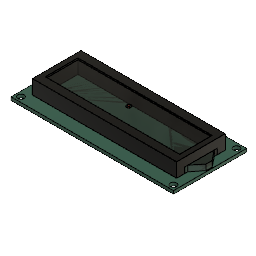
OTT Servo Tester Enclosure (Autodesk Fusion 360 archive; units mm, degrees)
design "1602 LCD Simplified Model"
Autodesk Fusion 360 part; units mm, degrees
sketch "LCD PCB" plane through (0, 0, 0) normal (0, 0, 1) x (1, 0, 0) in component "LCD PCB"
  line L0 (-40, 18) -> (40, 18)
  line L1 (40, 18) -> (40, -18)
  line L2 (40, -18) -> (-40, -18)
  line L3 (-40, -18) -> (-40, 18)
  line L4 (-40, 18) -> (40, -18) construction
  line L5 (40, 18) -> (-40, -18) construction
  line L6 (0, 1.75) -> (0, 22.5)
  line L7 (1.75, 0) -> (22.5, 0)
  point P0 (-37.5, 15.5)
  point P1 (37.5, 15.5)
  point P2 (-37.5, -15.5)
  point P3 (37.5, -15.5)
  point P4 (-32, 15.46)
  point P5 (-29.46, 15.46)
  point P6 (-26.92, 15.46)
  point P7 (-24.38, 15.46)
  point P8 (-21.84, 15.46)
  point P9 (-19.3, 15.46)
  point P10 (-16.76, 15.46)
  point P11 (-14.22, 15.46)
  point P12 (-11.68, 15.46)
  point P13 (-9.14, 15.46)
  point P14 (-6.6, 15.46)
  point P15 (-4.06, 15.46)
  point P16 (-1.52, 15.46)
  point P17 (1.02, 15.46)
  point P18 (3.56, 15.46)
  point P19 (6.1, 15.46)
  dimension "d1" = 80
  dimension "d2" = 36
  dimension "d3" = 2.5
  dimension "d4" = 2.5
  dimension "d5" = 8
  dimension "d6" = 2.54
  dimension "d9" = 2.54
  dimension "d10" = 0
  constraint horizontal L0
  constraint perpendicular L0 L1
  constraint parallel L0 L2
  constraint parallel L1 L3
  constraint coincident L4 origin
  constraint coincident L5 origin
  constraint symmetric P0 L6 P1
  constraint symmetric P0 L7 P2
  constraint symmetric P1 L7 P3
  measures "d1" distance of L1.end L2.end
  measures "d2" distance of L0.end L1.end
  measures "d3" distance of L0 P0
  measures "d4" distance of L3 P0
  measures "d5" distance of L3 P4
  measures "d6" distance of L0 P4
extrude "Extrude1" add sketch "LCD PCB" against normal blind 1.6 makes body 1 in component "LCD PCB"
hole "Hole1" at (-37.5, 15.5, 0) at (-37.5, -15.5, 0) at (37.5, -15.5, 0) at (37.5, 15.5, 0) direction (0, 0, -1) diameter 3.1 end up to surface (1.6 mm away) bodies 1 in component "LCD PCB"
hole "Hole2" at (6.1, 15.46, 0) at (3.56, 15.46, 0) at (1.02, 15.46, 0) at (-1.52, 15.46, 0) at (-4.06, 15.46, 0) at (-6.6, 15.46, 0) at (-9.14, 15.46, 0) at (-11.68, 15.46, 0) at (-14.22, 15.46, 0) at (-16.76, 15.46, 0) at (-19.3, 15.46, 0) at (-21.84, 15.46, 0) at (-24.38, 15.46, 0) at (-26.92, 15.46, 0) at (-29.46, 15.46, 0) at (-32, 15.46, 0) direction (0, 0, -1) diameter 1 depth 1.6 tip angle 180 bodies 1 in component "LCD PCB"
sketch "Bezel" plane through (0, 0, 0) normal (0, 0, 1) x (1, 0, 0) in component "LCD Bezel"
  line L0 (35.5, 12) -> (-35.5, 12)
  line L1 (-35.5, 12) -> (-35.5, -12)
  line L2 (-35.5, -12) -> (35.5, -12)
  line L3 (35.5, -12) -> (35.5, 12)
  line L4 (35.5, 12) -> (-35.5, -12) construction
  line L5 (-35.5, 12) -> (35.5, -12) construction
  line L6 (-33, 8) -> (33, 8)
  line L7 (33, 8) -> (33, -8)
  line L8 (33, -8) -> (-33, -8)
  line L9 (-33, -8) -> (-33, 8)
  line L10 (-33, 8) -> (33, -8) construction
  line L11 (33, 8) -> (-33, -8) construction
  dimension "d19" = 71
  dimension "d20" = 24
  dimension "d21" = 66
  dimension "d22" = 16
  constraint horizontal L0
  constraint perpendicular L0 L1
  constraint parallel L0 L2
  constraint parallel L1 L3
  constraint coincident L4 origin
  constraint coincident L5 origin
  constraint horizontal L6
  constraint perpendicular L6 L7
  constraint parallel L6 L8
  constraint parallel L7 L9
  constraint coincident L10 origin
  constraint coincident L11 origin
  measures "d19" distance of L1.end L2.end
  measures "d20" distance of L0.end L1.end
  measures "d21" distance of L7.end L8.end
  measures "d22" distance of L6.end L7.end
extrude "Extrude1'" add sketch "Bezel" along normal blind 7 separate body makes body 2 in component "LCD Bezel"
sketch "LCD Glass" plane through (0, 0, 7) normal (0, 0, 1) x (-1, 0, 0) in component "LCD Glass"
  line L0 (-33, 8) -> (33, 8)
  line L1 (33, 8) -> (33, -8)
  line L2 (33, -8) -> (-33, -8)
  line L3 (-33, -8) -> (-33, 8)
  line L4 (-35.5, 12) -> (-35.5, -12)
  line L5 (-35.5, -12) -> (35.5, -12)
  line L6 (35.5, -12) -> (35.5, 12)
  line L7 (35.5, 12) -> (-35.5, 12)
  line L8 (-35.5, 0) -> (-35.5, -6.5) construction
  line L9 (-35.5, -6.5) -> (-39.5, -1.5)
  line L10 (-39.5, -1.5) -> (-39.5, 0)
  line L11 (-1.75, 0) -> (-22.5, 0)
  line L12 (-40, -18) -> (-40, 18)
  line L13 (-35.5, 0) -> (-35.5, 6.5) construction
  line L14 (-35.5, 6.5) -> (-39.5, 1.5)
  line L15 (-39.5, 1.5) -> (-39.5, 0)
  line L16 (-35.5, -6.5) -> (-35.5, -8)
  line L17 (33, -8) -> (33, 8)
  line L18 (-35.5, 8) -> (-35.5, 6.5)
  line L19 (-35.5, 8) -> (33, 8)
  line L20 (33, -8) -> (-35.5, -8)
  line L21 (-35.5, -6.5) -> (-35.5, -8)
  circle A0 centre (0, 0) radius 1
  line L22 (0, -1) -> (0, 1)
  line L23 (1, 0) -> (-1, 0)
  circle A1 centre (0, 0) radius 1.1
  dimension "d25" = 6.5
  dimension "d26" = 1.5
  dimension "d27" = 0.5
  dimension "d130" = 2
  dimension "d131" = 2.2
  constraint midpoint L4 L8.start
  constraint coincident L4 L8.end
  constraint perpendicular L5 L8
  constraint perpendicular L10 L11
  constraint coincident L10.end L11
  constraint symmetric L8.start L11 L13.start
  constraint symmetric L8.end L11 L13.end
  constraint symmetric L9.end L11 L14.end
  constraint symmetric L10.end L11 L15.end
  constraint coincident L4 L16.end
  constraint perpendicular L2 L16
  constraint coincident L1.end L2.start
  constraint coincident L0.end L1.start
  constraint coincident L4 L18.start
  constraint parallel L4 L18
  constraint perpendicular L1 L19
  constraint parallel L16 L21
  constraint horizontal L20
  constraint coincident A0.centre A1.centre
  constraint coincident A0 L22.start
  constraint coincident A0 L22.end
  constraint vertical L22
  constraint coincident A0 L23.start
  constraint coincident A0 L23.end
  constraint perpendicular L22 L23
  constraint concentric A0 A1
  measures "d25" distance of L8.start L8.end
  measures "d26" distance of L9.end L10.end
  measures "d27" distance of L10 L12
  measures "d130" diameter of A0
  measures "d131" diameter of A1
extrude "Extrude1''" add sketch "LCD Glass" along normal blind 2.8 from surface at -7 separate body contours L0 L1 L2 L3 L17 L19 L20 | L3 L4 L16 L18 L19 L20 L21 | L4 L9 L10 L14 L15 | A0 L22 L23 | A0 L22 L23 | A0 L22 L23 | A0 L22 L23 | A1 makes body 3 in component "LCD Glass"
extrude "Extrude2" add sketch "LCD Glass" along normal up to surface (4.2 mm away) from surface at -4.2 contours L0 L1 L2 L3 L17 L19 L20 | A0 L22 L23 | A0 L22 L23 | A0 L22 L23 | A0 L22 L23 | A1 bodies 3 in component "LCD Glass"
extrude "Extrude3" cut sketch "LCD Glass" against normal blind 0.8 contours L0 L1 L2 L3 L17 L19 L20 | A0 L22 L23 | A0 L22 L23 | A0 L22 L23 | A0 L22 L23 | A1 bodies 3 in component "LCD Glass"
combine "Combine1" operation cut target body 2 tool bodies 3 keep tools in component "LCD Bezel"
extrude "Extrude1'''" add sketch "LCD Glass" against normal blind 0.1 separate body contours A0 L22 L23 | A0 L22 L23 | A1 picked at (0.6633, -0.0474) picked at (-0.6633, 0.0474) makes body 4
sketch "PCB Connector" plane through (0, 0, -1.6) normal (0, 0, -1) x (1, 0, 0) in component "PCB Connector"
  circle A0 centre (-29.46, -15.46) radius 0.5
  circle A1 centre (-24.38, -15.46) radius 0.5
  circle A2 centre (-19.3, -15.46) radius 0.5
  circle A3 centre (-14.22, -15.46) radius 0.5
  circle A4 centre (-9.14, -15.46) radius 0.5
  circle A5 centre (-4.06, -15.46) radius 0.5
  circle A6 centre (1.02, -15.46) radius 0.5
  circle A7 centre (6.1, -15.46) radius 0.5
  circle A8 centre (3.56, -15.46) radius 0.5
  circle A9 centre (-1.52, -15.46) radius 0.5
  circle A10 centre (-6.6, -15.46) radius 0.5
  circle A11 centre (-11.68, -15.46) radius 0.5
  circle A12 centre (-16.76, -15.46) radius 0.5
  circle A13 centre (-21.84, -15.46) radius 0.5
  circle A14 centre (-26.92, -15.46) radius 0.5
  circle A15 centre (-32, -15.46) radius 0.5
  circle A16 centre (37.5, 15.5) radius 1.55
  circle A17 centre (-37.5, -15.5) radius 1.55
  circle A18 centre (-37.5, 15.5) radius 1.55
  circle A19 centre (37.5, -15.5) radius 1.55
  line L0 (40, 18) -> (-40, 18)
  line L1 (-40, 18) -> (-40, -18)
  line L2 (-40, -18) -> (40, -18)
  line L3 (40, -18) -> (40, 18)
  line L4 (6.1, -15.46) -> (-32, -15.46) construction
  line L5 (7.37, -16.73) -> (-33.27, -16.73)
  line L6 (-33.27, -16.73) -> (-33.27, -14.19)
  line L7 (-33.27, -14.19) -> (7.37, -14.19)
  line L8 (7.37, -14.19) -> (7.37, -16.73)
  line L9 (6.425, -15.135) -> (5.775, -15.135)
  line L10 (5.775, -15.135) -> (5.775, -15.785)
  line L11 (5.775, -15.785) -> (6.425, -15.785)
  line L12 (6.425, -15.785) -> (6.425, -15.135)
  line L13 (6.425, -15.135) -> (5.775, -15.785) construction
  line L14 (5.775, -15.135) -> (6.425, -15.785) construction
  line L15 (3.235, -15.785) -> (3.885, -15.785)
  line L16 (3.235, -15.135) -> (3.235, -15.785)
  line L17 (3.885, -15.135) -> (3.235, -15.135)
  line L18 (3.885, -15.785) -> (3.885, -15.135)
  line L19 (0.695, -15.785) -> (1.345, -15.785)
  line L20 (0.695, -15.135) -> (0.695, -15.785)
  line L21 (1.345, -15.135) -> (0.695, -15.135)
  line L22 (1.345, -15.785) -> (1.345, -15.135)
  line L23 (-1.845, -15.785) -> (-1.195, -15.785)
  line L24 (-1.845, -15.135) -> (-1.845, -15.785)
  line L25 (-1.195, -15.135) -> (-1.845, -15.135)
  line L26 (-1.195, -15.785) -> (-1.195, -15.135)
  line L27 (-4.385, -15.785) -> (-3.735, -15.785)
  line L28 (-4.385, -15.135) -> (-4.385, -15.785)
  line L29 (-3.735, -15.135) -> (-4.385, -15.135)
  line L30 (-3.735, -15.785) -> (-3.735, -15.135)
  line L31 (-6.925, -15.785) -> (-6.275, -15.785)
  line L32 (-6.925, -15.135) -> (-6.925, -15.785)
  line L33 (-6.275, -15.135) -> (-6.925, -15.135)
  line L34 (-6.275, -15.785) -> (-6.275, -15.135)
  line L35 (-9.465, -15.785) -> (-8.815, -15.785)
  line L36 (-9.465, -15.135) -> (-9.465, -15.785)
  line L37 (-8.815, -15.135) -> (-9.465, -15.135)
  line L38 (-8.815, -15.785) -> (-8.815, -15.135)
  line L39 (-12.005, -15.785) -> (-11.355, -15.785)
  line L40 (-12.005, -15.135) -> (-12.005, -15.785)
  line L41 (-11.355, -15.135) -> (-12.005, -15.135)
  line L42 (-11.355, -15.785) -> (-11.355, -15.135)
  line L43 (-14.545, -15.785) -> (-13.895, -15.785)
  line L44 (-14.545, -15.135) -> (-14.545, -15.785)
  line L45 (-13.895, -15.135) -> (-14.545, -15.135)
  line L46 (-13.895, -15.785) -> (-13.895, -15.135)
  line L47 (-17.085, -15.785) -> (-16.435, -15.785)
  line L48 (-17.085, -15.135) -> (-17.085, -15.785)
  line L49 (-16.435, -15.135) -> (-17.085, -15.135)
  line L50 (-16.435, -15.785) -> (-16.435, -15.135)
  line L51 (-19.625, -15.785) -> (-18.975, -15.785)
  line L52 (-19.625, -15.135) -> (-19.625, -15.785)
  line L53 (-18.975, -15.135) -> (-19.625, -15.135)
  line L54 (-18.975, -15.785) -> (-18.975, -15.135)
  line L55 (-22.165, -15.785) -> (-21.515, -15.785)
  line L56 (-22.165, -15.135) -> (-22.165, -15.785)
  line L57 (-21.515, -15.135) -> (-22.165, -15.135)
  line L58 (-21.515, -15.785) -> (-21.515, -15.135)
  line L59 (-24.705, -15.785) -> (-24.055, -15.785)
  line L60 (-24.705, -15.135) -> (-24.705, -15.785)
  line L61 (-24.055, -15.135) -> (-24.705, -15.135)
  line L62 (-24.055, -15.785) -> (-24.055, -15.135)
  line L63 (-27.245, -15.785) -> (-26.595, -15.785)
  line L64 (-27.245, -15.135) -> (-27.245, -15.785)
  line L65 (-26.595, -15.135) -> (-27.245, -15.135)
  line L66 (-26.595, -15.785) -> (-26.595, -15.135)
  line L67 (-29.785, -15.785) -> (-29.135, -15.785)
  line L68 (-29.785, -15.135) -> (-29.785, -15.785)
  line L69 (-29.135, -15.135) -> (-29.785, -15.135)
  line L70 (-29.135, -15.785) -> (-29.135, -15.135)
  line L71 (-32.325, -15.785) -> (-31.675, -15.785)
  line L72 (-32.325, -15.135) -> (-32.325, -15.785)
  line L73 (-31.675, -15.135) -> (-32.325, -15.135)
  line L74 (-31.675, -15.785) -> (-31.675, -15.135)
  point P0 (-32, -15.46)
  point P1 (6.1, -15.46)
  dimension "d36" = 1.27
  dimension "d37" = 1.27
  dimension "d38" = 1.27
  dimension "d39" = 1.27
  dimension "d44" = 0.65
  dimension "d45" = 0.65
  dimension "d48" = -2.54
  dimension "d49" = 0
  constraint coincident P1 A7.centre
  constraint coincident P0 A15.centre
  constraint horizontal L5
  constraint vertical L6
  constraint horizontal L7
  constraint vertical L8
  constraint horizontal L9
  constraint perpendicular L9 L10
  constraint parallel L9 L11
  constraint parallel L10 L12
  constraint coincident L13 P1
  constraint coincident L14 P1
  measures "d36" distance of P1 L8
  measures "d37" distance of P0 L6
  measures "d38" distance of P1 L5
  measures "d39" distance of P1 L7
  measures "d44" distance of L10.end L11.end
  measures "d45" distance of L9.end L10.end
extrude "Extrude2'" add sketch "PCB Connector" along normal blind 6 and the other way blind 3 separate body contours L9 L10 L11 L12 | L15 L16 L17 L18 | L19 L20 L21 L22 | L23 L24 L25 L26 | L27 L28 L29 L30 | L31 L32 L33 L34 | L35 L36 L37 L38 | L39 L40 L41 L42 | L43 L44 L45 L46 | L47 L48 L49 L50 | L51 L52 L53 L54 | L55 L56 L57 L58 | L59 L60 L61 L62 | L63 L64 L65 L66 | L67 L68 L69 L70 | L71 L72 L73 L74 makes body 5 at (-27.245, 15.3517, -1.6) makes body 6 at (-17.085, 15.3517, -1.6) makes body 7 at (-6.925, 15.3517, -1.6) makes body 8 at (3.235, 15.3517, -1.6) makes body 9 at (0.695, 15.3517, -1.6) makes body 10 at (-9.465, 15.3517, -1.6) makes body 11 at (-19.625, 15.3517, -1.6) makes body 12 at (-29.3517, 15.135, -1.6) makes body 13 at (-24.2717, 15.135, -1.6) makes body 14 at (-14.545, 15.3517, -1.6) makes body 15 at (-4.385, 15.3517, -1.6) makes body 16 at (6.425, 15.5683, -1.6) makes body 17 at (-1.845, 15.3517, -1.6) makes body 18 at (-12.005, 15.3517, -1.6) makes body 19 at (-22.165, 15.3517, -1.6) makes body 20 at (-32.325, 15.3517, -1.6) in component "PCB Connector"
extrude "Extrude1''''" add sketch "PCB Connector" along normal blind 2.54 separate body contours A0 | A1 | A2 | A3 | A4 | A5 | A6 | A7 | A8 | A9 | A10 | A11 | A12 | A13 | A14 | A15 | L5 L6 L7 L8 makes body 21 in component "PCB Connector"
sketch "I2C PCB" plane through (0, 0, -4.14) normal (0, 0, -1) x (1, 0, 0) in component "I2C PCB"
  line L0 (7.37, -14.19) -> (-33.27, -14.19) construction
  line L1 (-33.27, -14.19) -> (-33.27, -16.73)
  line L2 (-33.27, -16.73) -> (7.37, -16.73)
  line L3 (7.37, -16.73) -> (7.37, -14.19)
  line L4 (8.64, -16.73) -> (-34.54, -16.73)
  line L5 (-34.54, -16.73) -> (-34.54, 2.27)
  line L6 (-34.54, 2.27) -> (8.64, 2.27)
  line L7 (8.64, 2.27) -> (8.64, -16.73)
  line L8 (8.64, -7.23) -> (-34.54, -7.23) construction
  line L9 (-26.64, -5.43) -> (-20.04, -5.43)
  line L10 (-20.04, -5.43) -> (-20.04, -12.23)
  line L11 (-20.04, -12.23) -> (-26.64, -12.23)
  line L12 (-26.64, -12.23) -> (-26.64, -5.43)
  line L13 (-7.26, -13.43) -> (-14.36, -13.43)
  line L14 (-14.36, -13.43) -> (-14.36, -3.43)
  line L15 (-14.36, -3.43) -> (-7.26, -3.43)
  line L16 (-7.26, -3.43) -> (-7.26, -13.43)
  line L17 (-13.895, -15.135) -> (-13.895, -15.785)
  line L18 (-13.895, -15.785) -> (-14.545, -15.785)
  line L19 (-14.545, -15.785) -> (-14.545, -15.135)
  line L20 (-14.545, -15.135) -> (-13.895, -15.135)
  line L21 (-16.435, -15.135) -> (-16.435, -15.785)
  line L22 (-16.435, -15.785) -> (-17.085, -15.785)
  line L23 (-17.085, -15.785) -> (-17.085, -15.135)
  line L24 (-17.085, -15.135) -> (-16.435, -15.135)
  line L25 (-18.975, -15.135) -> (-18.975, -15.785)
  line L26 (-18.975, -15.785) -> (-19.625, -15.785)
  line L27 (-19.625, -15.785) -> (-19.625, -15.135)
  line L28 (-19.625, -15.135) -> (-18.975, -15.135)
  line L29 (-21.515, -15.135) -> (-21.515, -15.785)
  line L30 (-21.515, -15.785) -> (-22.165, -15.785)
  line L31 (-22.165, -15.785) -> (-22.165, -15.135)
  line L32 (-22.165, -15.135) -> (-21.515, -15.135)
  line L33 (-11.355, -15.135) -> (-11.355, -15.785)
  line L34 (-11.355, -15.785) -> (-12.005, -15.785)
  line L35 (-12.005, -15.785) -> (-12.005, -15.135)
  line L36 (-12.005, -15.135) -> (-11.355, -15.135)
  line L37 (-8.815, -15.135) -> (-8.815, -15.785)
  line L38 (-8.815, -15.785) -> (-9.465, -15.785)
  line L39 (-9.465, -15.785) -> (-9.465, -15.135)
  line L40 (-9.465, -15.135) -> (-8.815, -15.135)
  line L41 (-6.275, -15.135) -> (-6.275, -15.785)
  line L42 (-6.275, -15.785) -> (-6.925, -15.785)
  line L43 (-6.925, -15.785) -> (-6.925, -15.135)
  line L44 (-6.925, -15.135) -> (-6.275, -15.135)
  line L45 (-3.735, -15.135) -> (-3.735, -15.785)
  line L46 (-3.735, -15.785) -> (-4.385, -15.785)
  line L47 (-4.385, -15.785) -> (-4.385, -15.135)
  line L48 (-4.385, -15.135) -> (-3.735, -15.135)
  line L49 (-1.195, -15.135) -> (-1.195, -15.785)
  line L50 (-1.195, -15.785) -> (-1.845, -15.785)
  line L51 (-1.845, -15.785) -> (-1.845, -15.135)
  line L52 (-1.845, -15.135) -> (-1.195, -15.135)
  line L53 (1.345, -15.135) -> (1.345, -15.785)
  line L54 (1.345, -15.785) -> (0.695, -15.785)
  line L55 (0.695, -15.785) -> (0.695, -15.135)
  line L56 (0.695, -15.135) -> (1.345, -15.135)
  line L57 (3.885, -15.135) -> (3.885, -15.785)
  line L58 (3.885, -15.785) -> (3.235, -15.785)
  line L59 (3.235, -15.785) -> (3.235, -15.135)
  line L60 (3.235, -15.135) -> (3.885, -15.135)
  line L61 (6.425, -15.135) -> (6.425, -15.785)
  line L62 (6.425, -15.785) -> (5.775, -15.785)
  line L63 (5.775, -15.785) -> (5.775, -15.135)
  line L64 (5.775, -15.135) -> (6.425, -15.135)
  line L65 (-26.595, -15.135) -> (-26.595, -15.785)
  line L66 (-26.595, -15.785) -> (-27.245, -15.785)
  line L67 (-27.245, -15.785) -> (-27.245, -15.135)
  line L68 (-27.245, -15.135) -> (-26.595, -15.135)
  line L69 (-31.675, -15.135) -> (-31.675, -15.785)
  line L70 (-31.675, -15.785) -> (-32.325, -15.785)
  line L71 (-32.325, -15.785) -> (-32.325, -15.135)
  line L72 (-32.325, -15.135) -> (-31.675, -15.135)
  line L73 (-29.135, -15.135) -> (-29.135, -15.785)
  line L74 (-29.135, -15.785) -> (-29.785, -15.785)
  line L75 (-29.785, -15.785) -> (-29.785, -15.135)
  line L76 (-29.785, -15.135) -> (-29.135, -15.135)
  line L77 (-24.055, -15.135) -> (-24.055, -15.785)
  line L78 (-24.055, -15.785) -> (-24.705, -15.785)
  line L79 (-24.705, -15.785) -> (-24.705, -15.135)
  line L80 (-24.705, -15.135) -> (-24.055, -15.135)
  circle A0 centre (6.1, -15.46) radius 0.5
  circle A1 centre (6.1, -15.46) radius 0.5
  circle A2 centre (3.56, -15.46) radius 0.5
  circle A3 centre (1.02, -15.46) radius 0.5
  circle A4 centre (-1.52, -15.46) radius 0.5
  circle A5 centre (-4.06, -15.46) radius 0.5
  circle A6 centre (-6.6, -15.46) radius 0.5
  circle A7 centre (-9.14, -15.46) radius 0.5
  circle A8 centre (-11.68, -15.46) radius 0.5
  circle A9 centre (-14.22, -15.46) radius 0.5
  circle A10 centre (-16.76, -15.46) radius 0.5
  circle A11 centre (-19.3, -15.46) radius 0.5
  circle A12 centre (-21.84, -15.46) radius 0.5
  circle A13 centre (-24.38, -15.46) radius 0.5
  circle A14 centre (-26.92, -15.46) radius 0.5
  circle A15 centre (-29.46, -15.46) radius 0.5
  circle A16 centre (-32, -15.46) radius 0.5
  point P0 (7.37, -7.23)
  point P1 (7.37, -9.77)
  point P2 (-33.27, -3.23)
  point P3 (-33.27, -5.77)
  point P4 (-33.27, -8.31)
  point P5 (-33.27, -10.85)
  dimension "d54" = 1.27
  dimension "d55" = 1.27
  dimension "d56" = 19
  dimension "d57" = 2.54
  dimension "d58" = 1.27
  dimension "d59" = 1.27
  dimension "d60" = 5.5
  dimension "d63" = 0
  dimension "d64" = -2.54
  dimension "d70" = 6.6
  dimension "d71" = 6.8
  dimension "d73" = 14.5
  dimension "d74" = 14.5
  dimension "d75" = 7.1
  dimension "d76" = 10
  dimension "d77" = 23
  dimension "d78" = 15.7
  dimension "d135" = 1
  dimension "d138" = -2.54
  dimension "d139" = 0
  constraint horizontal L4
  constraint vertical L5
  constraint horizontal L6
  constraint vertical L7
  constraint collinear L2 L4
  constraint midpoint L7 L8.start
  constraint midpoint L5 L8.end
  constraint coincident L8 P0
  constraint vertical P0 P1
  constraint horizontal L9
  constraint vertical L10
  constraint horizontal L11
  constraint vertical L12
  constraint horizontal L13
  constraint vertical L14
  constraint horizontal L15
  constraint vertical L16
  constraint concentric A0 A1
  measures "d54" distance of L3 L7
  measures "d55" distance of L1 L5
  measures "d56" distance of L4 L6
  measures "d57" distance of P0 P1
  measures "d58" distance of L7 P0
  measures "d59" distance of L5 P2
  measures "d60" distance of L6 P2
  measures "d70" distance of L9.start L9.end
  measures "d71" distance of L9.start L11.end
  measures "d73" distance of L5 L10.end
  measures "d74" distance of L6 L10.end
  measures "d75" distance of L13.start L13.end
  measures "d76" distance of L13.start L15.end
  measures "d77" distance of L7 L14
  measures "d78" distance of L6 L13
  measures "d135" diameter of A0
extrude "Extrude1'''''" add sketch "I2C PCB" along normal blind 1.6 separate body contours L2 L4 L5 L6 L7 | L9 L10 L11 L12 | L13 L14 L15 L16 makes body 22 in component "I2C PCB"
extrude "Extrude2''" add sketch "I2C PCB" along normal blind 3 from surface at 1.6 separate body contours L13 L14 L15 L16 makes body 23 in component "I2C PCB"
extrude "Extrude3'" add sketch "I2C PCB" along normal blind 5.1 from surface at 1.6 separate body contours L9 L10 L11 L12 makes body 24 in component "I2C PCB"
hole "Hole1'" at (7.37, 7.23, -4.14) at (7.37, 9.77, -4.14) at (-33.27, 3.23, -4.14) at (-33.27, 5.77, -4.14) at (-33.27, 8.31, -4.14) at (-33.27, 10.85, -4.14) direction (0, 0, -1) diameter 1 end up to surface (1.6 mm away) bodies 22 in component "I2C PCB"
sketch "Connector" plane through (0, 0, -5.74) normal (0, 0, -1) x (1, 0, 0) in component "I2C Connectors"
  circle A0 centre (-33.27, -8.31) radius 0.5
  circle A1 centre (-33.27, -3.23) radius 0.5
  circle A2 centre (7.37, -7.23) radius 0.5
  circle A3 centre (7.37, -9.77) radius 0.5
  circle A4 centre (-33.27, -5.77) radius 0.5
  circle A5 centre (-33.27, -10.85) radius 0.5
  line L0 (8.64, 2.27) -> (-34.54, 2.27)
  line L1 (-34.54, 2.27) -> (-34.54, -16.73)
  line L2 (-34.54, -16.73) -> (8.64, -16.73)
  line L3 (8.64, -16.73) -> (8.64, 2.27)
  line L4 (6.1, -11.04) -> (8.64, -11.04)
  line L5 (8.64, -11.04) -> (8.64, -5.96)
  line L6 (8.64, -5.96) -> (6.1, -5.96)
  line L7 (6.1, -5.96) -> (6.1, -11.04)
  line L8 (-32, -12.12) -> (-34.54, -12.12)
  line L9 (-34.54, -12.12) -> (-34.54, -1.96)
  line L10 (-34.54, -1.96) -> (-32, -1.96)
  line L11 (-32, -1.96) -> (-32, -12.12)
  line L12 (7.695, -10.095) -> (7.045, -10.095)
  line L13 (7.045, -10.095) -> (7.045, -9.445)
  line L14 (7.045, -9.445) -> (7.695, -9.445)
  line L15 (7.695, -9.445) -> (7.695, -10.095)
  line L16 (7.695, -10.095) -> (7.045, -9.445) construction
  line L17 (7.045, -10.095) -> (7.695, -9.445) construction
  line L18 (7.695, -7.555) -> (7.045, -7.555)
  line L19 (7.045, -7.555) -> (7.045, -6.905)
  line L20 (7.045, -6.905) -> (7.695, -6.905)
  line L21 (7.695, -6.905) -> (7.695, -7.555)
  line L22 (7.695, -7.555) -> (7.045, -6.905) construction
  line L23 (7.045, -7.555) -> (7.695, -6.905) construction
  line L24 (-33.595, -11.175) -> (-32.945, -11.175)
  line L25 (-32.945, -11.175) -> (-32.945, -10.525)
  line L26 (-32.945, -10.525) -> (-33.595, -10.525)
  line L27 (-33.595, -10.525) -> (-33.595, -11.175)
  line L28 (-33.595, -11.175) -> (-32.945, -10.525) construction
  line L29 (-32.945, -11.175) -> (-33.595, -10.525) construction
  line L30 (-32.945, -7.985) -> (-33.595, -7.985)
  line L31 (-33.595, -7.985) -> (-33.595, -8.635)
  line L32 (-33.595, -8.635) -> (-32.945, -8.635)
  line L33 (-32.945, -8.635) -> (-32.945, -7.985)
  line L34 (-32.945, -5.445) -> (-33.595, -5.445)
  line L35 (-33.595, -5.445) -> (-33.595, -6.095)
  line L36 (-33.595, -6.095) -> (-32.945, -6.095)
  line L37 (-32.945, -6.095) -> (-32.945, -5.445)
  line L38 (-32.945, -2.905) -> (-33.595, -2.905)
  line L39 (-33.595, -2.905) -> (-33.595, -3.555)
  line L40 (-33.595, -3.555) -> (-32.945, -3.555)
  line L41 (-32.945, -3.555) -> (-32.945, -2.905)
  circle A6 centre (-24.38, -15.46) radius 0.5
  circle A7 centre (-26.92, -15.46) radius 0.5
  circle A8 centre (-9.14, -15.46) radius 0.5
  circle A9 centre (-21.84, -15.46) radius 0.5
  circle A10 centre (-32, -15.46) radius 0.5
  circle A11 centre (-29.46, -15.46) radius 0.5
  circle A12 centre (-11.68, -15.46) radius 0.5
  circle A13 centre (-14.22, -15.46) radius 0.5
  circle A14 centre (-16.76, -15.46) radius 0.5
  circle A15 centre (-19.3, -15.46) radius 0.5
  circle A16 centre (-6.6, -15.46) radius 0.5
  circle A17 centre (-4.06, -15.46) radius 0.5
  circle A18 centre (-1.52, -15.46) radius 0.5
  circle A19 centre (1.02, -15.46) radius 0.5
  circle A20 centre (3.56, -15.46) radius 0.5
  circle A21 centre (6.1, -15.46) radius 0.5
  point P0 (7.37, -9.77)
  point P1 (7.37, -7.23)
  point P2 (-33.27, -10.85)
  dimension "d85" = 1.27
  dimension "d86" = 1.27
  dimension "d87" = 2.54
  dimension "d88" = 1.27
  dimension "d89" = 1.27
  dimension "d90" = 2.54
  dimension "d91" = 0.65
  dimension "d92" = 0.65
  dimension "d93" = 0.65
  dimension "d94" = 0.65
  dimension "d97" = 0.65
  dimension "d98" = 0.65
  dimension "d101" = 0
  dimension "d102" = 2.54
  constraint horizontal L4
  constraint vertical L5
  constraint horizontal L6
  constraint vertical L7
  constraint horizontal L8
  constraint vertical L9
  constraint horizontal L10
  constraint vertical L11
  constraint collinear L1 L9
  constraint collinear L3 L5
  constraint horizontal L12
  constraint perpendicular L12 L13
  constraint parallel L12 L14
  constraint parallel L13 L15
  constraint coincident L16 P0
  constraint coincident L17 P0
  constraint coincident P0 A3.centre
  constraint horizontal L18
  constraint perpendicular L18 L19
  constraint parallel L18 L20
  constraint parallel L19 L21
  constraint coincident L22 P1
  constraint coincident L23 P1
  constraint coincident P1 A2.centre
  constraint horizontal L24
  constraint perpendicular L24 L25
  constraint parallel L24 L26
  constraint parallel L25 L27
  constraint coincident L28 P2
  constraint coincident L29 P2
  constraint coincident P2 A5.centre
  measures "d85" distance of P0 L4
  measures "d86" distance of P1 L6
  measures "d87" distance of L5 L7
  measures "d88" distance of P2 L8
  measures "d89" distance of A1.centre L10
  measures "d90" distance of L9 L11
  measures "d91" distance of L13.end L14.end
  measures "d92" distance of L12.end L13.end
  measures "d93" distance of L19.end L20.end
  measures "d94" distance of L18.end L19.end
  measures "d97" distance of L25.end L26.end
  measures "d98" distance of L24.end L25.end
extrude "Extrude1''''''" add sketch "Connector" along normal blind 2.54 separate body contours A0 | A1 | A2 | A3 | A4 | A5 | L3 L4 L5 L6 L7 | L1 L8 L9 L10 L11 makes body 25 at (8.64, 9.3467, -6.5867) makes body 26 at (-34.54, 5.3467, -6.5867) in component "I2C Connectors"
sketch "Pins" plane through (0, 5.96, 0) normal (0, -1, 0) x (1, 0, 0) in component "I2C Connectors"
  line L0 (8.64, -5.74) -> (6.1, -5.74)
  line L1 (6.1, -5.74) -> (6.1, -8.28)
  line L2 (6.1, -8.28) -> (8.64, -8.28)
  line L3 (8.64, -8.28) -> (8.64, -5.74)
  line L4 (7.37, -10.74) -> (7.37, -3.14)
  line L5 (8.64, -4.14) -> (-34.54, -4.14)
  line L6 (-34.54, -4.14) -> (-34.54, -5.74)
  line L7 (-34.54, -5.74) -> (8.64, -5.74)
  line L8 (8.64, -5.74) -> (8.64, -4.14)
  line L9 (8.37, -11.74) -> (14.87, -11.74)
  arc A0 (7.37, -10.74) -> (8.37, -11.74) centre (8.37, -10.74) ccw
  point P0 (7.37, -8.28)
  dimension "d103" = 1
  dimension "d104" = 7.5
  dimension "d105" = 6
  dimension "d106" = 1
  constraint vertical L4
  constraint perpendicular L4 L9
  constraint midpoint L2 P0
  constraint coincident L4 P0
  constraint tangent L9 A0
  constraint tangent L4 A0
  measures "d103" vertical distance of L4.end L5.start
  measures "d104" distance of L4 L9.end
  measures "d105" distance of L0 L9
  measures "d106" radius of A0
pipe "Pipe1" add square section size 0.65 path "Pins" along L9 A0 L4 separate body makes body 27 in component "I2C Connectors"
ref_plane "WorkPlane1" through (-12.95, 7.23, -4.94) normal (1, 0, 0) x (0, -1, 0) in component "I2C Connectors"
mirror "Mirror1" about plane through (-12.95, 7.23, -4.94) normal (1, 0, 0) of bodies 27 makes body 28 in component "I2C Connectors"
move_body "Move3" bodies 28 to x (1, 0, 0) y (0, 1, 0) z (0, 0, 1) at (0, -2.75, 0) in component "I2C Connectors"
move_body "Move1" bodies 27 to x (1, 0, 0) y (0, 1, 0) z (0, 0, 1) at (0, 1.27, 0) in component "I2C Connectors"
pattern_linear "R-Pattern1" count 2 spacing 2.54 along (0, 1, 0) of bodies 27 makes body 29 in component "I2C Connectors"
pattern_linear "R-Pattern2" count 4 spacing 2.54 along (0, 1, 0) of bodies 28 makes body 30 at (-32.945, 5.6417, -8.2067) makes body 31 at (-32.945, 8.1817, -8.2067) makes body 32 at (-32.945, 10.7217, -8.2067) in component "I2C Connectors"
copy_body "CutPasteBodies1" bodies 4 removing the originals makes body 33 in component "LCD Glass"
component "LCD PCB" placed x (1, 0, 0) y (0, 1, 0) z (0, 0, 1) at (0, 0, 0)
component "LCD Bezel" placed x (1, 0, 0) y (0, 1, 0) z (0, 0, 1) at (0, 0, 0)
component "LCD Glass" placed x (1, 0, 0) y (0, 1, 0) z (0, 0, 1) at (0, 0, 0)
component "PCB Connector" placed x (1, 0, 0) y (0, 1, 0) z (0, 0, 1) at (0, 0, 0)
component "I2C PCB" placed x (1, 0, 0) y (0, 1, 0) z (0, 0, 1) at (0, 0, 0)
component "I2C Connectors" placed x (1, 0, 0) y (0, 1, 0) z (0, 0, 1) at (0, 0, 0)
equation "d37 = d36"
equation "d38 = d36"
equation "d39 = d36"
named bodies: "LCD PCB", "Bezel", "Glass", "LCD Header", "PCB", "IC", "Pot", "LED Jumper", "I2C Header"

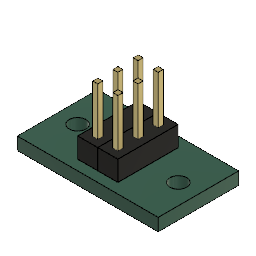
design "Power Header"
Autodesk Fusion 360 part; units mm, degrees
sketch "PCB" plane through (0, 0, 0) normal (0, 0, 1) x (1, 0, 0)
  line L0 (-8.89, 5.08) -> (8.89, 5.08)
  line L1 (8.89, 5.08) -> (8.89, -5.08)
  line L2 (8.89, -5.08) -> (-8.89, -5.08)
  line L3 (-8.89, -5.08) -> (-8.89, 5.08)
  line L4 (-8.89, 5.08) -> (8.89, -5.08) construction
  line L5 (8.89, 5.08) -> (-8.89, -5.08) construction
  line L6 (1.75, 0) -> (22.5, 0)
  circle A0 centre (-6.35, 0) radius 1.05
  line L7 (0, 1.75) -> (0, 22.5)
  circle A1 centre (6.35, 0) radius 1.05
  point P0 (-1.27, -2.54)
  point P1 (1.27, -2.54)
  point P2 (-1.27, 0)
  point P3 (1.27, 0)
  point P4 (-1.27, 2.54)
  point P5 (1.27, 2.54)
  dimension "d3" = 2.54
  dimension "d4" = 2.54
  dimension "d5" = 1.27
  dimension "d7" = 2.54
  dimension "d8" = 2.1
  dimension "d9" = 5.08
  dimension "d10" = 2.54
  dimension "d37" = 10.16
  dimension "d38" = 17.78
  constraint horizontal L0
  constraint perpendicular L0 L1
  constraint parallel L0 L2
  constraint parallel L1 L3
  constraint coincident L4 origin
  constraint coincident L5 origin
  constraint coincident P2 L6
  constraint symmetric A0 L7 A1
  measures "d5" distance of origin P2
  measures "d7" distance of L0 P4
  measures "d8" diameter of A0
  measures "d9" distance of P2 A0.centre
  measures "d10" distance of L3 A0.centre
  measures "d37" distance of L0.start L2.end
  measures "d38" distance of L0.start L0.end
extrude "Extrude1" add sketch "PCB" along normal blind 1.6 makes body 1
hole "Hole1" at (-1.27, 2.54, 0) at (1.27, 2.54, 0) at (1.27, 0, 0) at (-1.27, 0, 0) at (-1.27, -2.54, 0) at (1.27, -2.54, 0) direction (0, 0, 1) diameter 1 end up to surface (1.6 mm away) bodies 1
sketch "Header Pins" plane through (0, 0, 1.6) normal (0, 0, 1) x (-1, 0, 0) in component "Header"
  circle A0 centre (1.27, 2.54) radius 0.5 construction
  circle A1 centre (-1.27, 0) radius 0.5
  circle A2 centre (1.27, -2.54) radius 0.5 construction
  circle A3 centre (-1.27, -2.54) radius 0.5
  circle A4 centre (1.27, 0) radius 0.5 construction
  circle A5 centre (-1.27, 2.54) radius 0.5
  circle A6 centre (6.35, 0) radius 1.05
  circle A7 centre (-6.35, 0) radius 1.05
  line L0 (8.89, 5.08) -> (-8.89, 5.08)
  line L1 (-8.89, 5.08) -> (-8.89, -5.08)
  line L2 (-8.89, -5.08) -> (8.89, -5.08)
  line L3 (8.89, -5.08) -> (8.89, 5.08)
  line L4 (2.54, -3.81) -> (0, -3.81)
  line L5 (0, -3.81) -> (0, 3.81)
  line L6 (0, 3.81) -> (2.54, 3.81)
  line L7 (2.54, 3.81) -> (2.54, -3.81)
  line L8 (1.595, -2.215) -> (0.945, -2.215)
  line L9 (0.945, -2.215) -> (0.945, -2.865)
  line L10 (0.945, -2.865) -> (1.595, -2.865)
  line L11 (1.595, -2.865) -> (1.595, -2.215)
  line L12 (1.595, -2.215) -> (0.945, -2.865) construction
  line L13 (0.945, -2.215) -> (1.595, -2.865) construction
  point P0 (1.27, -2.54)
  dimension "d16" = 1.27
  dimension "d17" = 1.27
  dimension "d18" = 1.27
  dimension "d19" = 1.27
  dimension "d20" = 0.65
  dimension "d21" = 0.65
  constraint horizontal L4
  constraint vertical L5
  constraint horizontal L6
  constraint vertical L7
  constraint horizontal L8
  constraint perpendicular L8 L9
  constraint parallel L8 L10
  constraint parallel L9 L11
  constraint coincident L12 P0
  constraint coincident L13 P0
  constraint coincident P0 A2.centre
  measures "d16" distance of A0.centre L5
  measures "d17" distance of A0.centre L7
  measures "d18" distance of P0 L4
  measures "d19" distance of A0.centre L6
  measures "d20" distance of L8.end L9.end
  measures "d21" distance of L8.start L8.end
extrude "Extrude1'" add sketch "Header Pins" along normal blind 2.54 separate body contours L4 L5 L6 L7 | L8 L9 L10 L11 makes body 2 in component "Header"
extrude "Extrude2" add sketch "Header Pins" along normal blind 8.54 and the other way blind 3 separate body contours L8 L9 L10 L11 makes body 3 in component "Header"
pattern_linear "R-Pattern1" count 2 spacing 2.54 along (1, 0, 0) count 3 spacing 2.54 along (0, -1, 0) of bodies 3 makes body 4 at (1.3783, 2.215, 6.2933) makes body 5 at (-1.1617, -0.325, 6.2933) makes body 6 at (1.3783, -0.325, 6.2933) makes body 7 at (-1.1617, -2.865, 6.2933) makes body 8 at (1.3783, -2.865, 6.2933) in component "Header"
pattern_linear "R-Pattern2" count 2 spacing 2.54 along (1, 0, 0) of bodies 2 makes body 9 in component "Header"
copy_body "Body->Comp1" bodies 1 removing the originals makes body 10 in component "PCB"
component "Header" placed x (1, 0, 0) y (0, 1, 0) z (0, 0, 1) at (0, 0, 0)
component "PCB" placed x (1, 0, 0) y (0, 1, 0) z (0, 0, 1) at (0, 0, 0)
named bodies: "PCB", "Header Plastic", "Header Pin", "Header Pin (1)", "Header Pin (2)", "Header Pin (3)", "Header Pin (4)", "Header Pin (5)", "Header Plastic (1)"

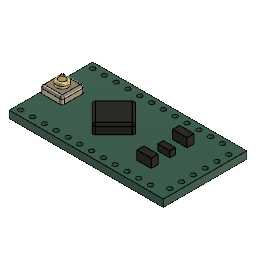
design "Arduino Pro Micro Simplified Model"
Autodesk Fusion 360 part; units mm, degrees
sketch "Layout" plane through (0, 0, 0) normal (0, 0, 1) x (1, 0, 0)
  line L0 (-16.6, 9) -> (16.6, 9)
  line L1 (16.6, 9) -> (16.6, -9)
  line L2 (16.6, -9) -> (-16.6, -9)
  line L3 (-16.6, -9) -> (-16.6, 9)
  line L4 (-16.6, 9) -> (16.6, -9) construction
  line L5 (16.6, 9) -> (-16.6, -9) construction
  line L6 (-16.6, 2.45) -> (-11.7, 2.45)
  line L7 (-11.7, 2.45) -> (-11.7, -2.45)
  line L8 (-11.7, -2.45) -> (-16.6, -2.45)
  line L9 (-16.6, -2.45) -> (-16.6, 2.45)
  line L10 (-3.0331, 4.6669) -> (-7.7, 0)
  line L11 (-7.7, 0) -> (-3.0331, -4.6669)
  line L12 (1.75, 0) -> (22.5, 0)
  circle A0 centre (-14.15, 0) radius 1.25
  line L13 (-16.6, 0) -> (-11.7, 0) construction
  line L14 (-3.0331, 4.6669) -> (1.6338, 0)
  line L15 (1.6338, 0) -> (-3.0331, -4.6669)
  line L16 (7, 0.6) -> (9.6, 0.6)
  line L17 (9.6, 0.6) -> (9.6, -0.6)
  line L18 (9.6, -0.6) -> (7, -0.6)
  line L19 (7, -0.6) -> (7, 0.6)
  line L20 (6.5, 4.6) -> (9.6, 4.6)
  line L21 (9.6, 4.6) -> (9.6, 3.1)
  line L22 (9.6, 3.1) -> (6.5, 3.1)
  line L23 (6.5, 3.1) -> (6.5, 4.6)
  line L24 (6.5, -4.6) -> (9.6, -4.6)
  line L25 (6.5, -3.1) -> (6.5, -4.6)
  line L26 (9.6, -3.1) -> (6.5, -3.1)
  line L27 (9.6, -4.6) -> (9.6, -3.1)
  point P0 (-16.6, 0)
  point P1 (-14.15, 0)
  point P2 (-15.33, -7.73)
  point P3 (-12.79, -7.73)
  point P4 (-10.25, -7.73)
  point P5 (-7.71, -7.73)
  point P6 (-5.17, -7.73)
  point P7 (-2.63, -7.73)
  point P8 (-0.09, -7.73)
  point P9 (2.45, -7.73)
  point P10 (4.99, -7.73)
  point P11 (7.53, -7.73)
  point P12 (10.07, -7.73)
  point P13 (12.61, -7.73)
  point P14 (-15.33, 7.73)
  point P15 (-12.79, 7.73)
  point P16 (-10.25, 7.73)
  point P17 (-7.71, 7.73)
  point P18 (-5.17, 7.73)
  point P19 (-2.63, 7.73)
  point P20 (-0.09, 7.73)
  point P21 (2.45, 7.73)
  point P22 (4.99, 7.73)
  point P23 (7.53, 7.73)
  point P24 (10.07, 7.73)
  point P25 (12.61, 7.73)
  point P26 (15.33, -6.35)
  point P27 (15.33, -3.81)
  point P28 (15.33, -1.27)
  point P29 (15.33, 1.27)
  point P30 (15.33, 3.81)
  point P31 (15.33, 6.35)
  point P32 (7, 0)
  dimension "d1" = 33.2
  dimension "d2" = 18
  dimension "d3" = 4.9
  dimension "d4" = 4.9
  dimension "d5" = 2.5
  dimension "d6" = 1.27
  dimension "d7" = 1.27
  dimension "d10" = 2.54
  dimension "d11" = 0
  dimension "d12" = 1.27
  dimension "d13" = 2.65
  dimension "d16" = 0
  dimension "d17" = 2.54
  dimension "d18" = 2.76
  dimension "d19" = 6.6
  dimension "d21" = 4
  dimension "d22" = 6.6
  dimension "d41" = 3.1
  dimension "d42" = 1.5
  dimension "d43" = 2.6
  dimension "d44" = 1.2
  dimension "d45" = 5.9
  dimension "d46" = 10.1
  constraint horizontal L0
  constraint perpendicular L0 L1
  constraint parallel L0 L2
  constraint parallel L1 L3
  constraint coincident L4 origin
  constraint coincident L5 origin
  constraint horizontal L6
  constraint vertical L7
  constraint horizontal L8
  constraint vertical L9
  constraint perpendicular L10 L11
  constraint midpoint L9 P0
  constraint coincident P0 L12
  constraint collinear L3 L9
  constraint coincident P0 L13.start
  constraint midpoint L7 L13.end
  constraint midpoint L13 P1
  constraint coincident P1 A0.centre
  constraint symmetric L12 P2 P14
  constraint symmetric L12 P3 P15
  constraint symmetric L12 P4 P16
  constraint symmetric L12 P5 P17
  constraint symmetric L12 P6 P18
  constraint symmetric L12 P7 P19
  constraint symmetric L12 P8 P20
  constraint symmetric L12 P9 P21
  constraint symmetric L12 P10 P22
  constraint symmetric L12 P11 P23
  constraint symmetric L12 P12 P24
  constraint symmetric L12 P13 P25
  constraint coincident L10.end L12
  constraint perpendicular L10 L14
  constraint perpendicular L11 L15
  constraint coincident L12 L14.end
  constraint horizontal L16
  constraint vertical L17
  constraint horizontal L18
  constraint vertical L19
  constraint horizontal L20
  constraint vertical L21
  constraint horizontal L22
  constraint vertical L23
  constraint collinear L17 L21
  constraint symmetric L12 L20.start L24.start
  constraint symmetric L12 L20.end L24.end
  constraint symmetric L12 L21.end L26.start
  constraint symmetric L12 L22.end L25.start
  constraint midpoint L19 P32
  constraint coincident L12 P32
  measures "d1" distance of L1.end L2.end
  measures "d2" distance of L0.end L1.end
  measures "d3" distance of L6.start L6.end
  measures "d4" distance of L6.start L8.end
  measures "d5" diameter of A0
  measures "d6" distance of L3 P2
  measures "d7" distance of L2 P2
  measures "d12" distance of L1 P26
  measures "d13" distance of L2 P26
  measures "d19" distance of L10.start L10.end
  measures "d21" distance of L10.end L13.end
  measures "d22" distance of L10 L15
  measures "d41" distance of L20.start L20.end
  measures "d42" distance of L20.end L21.end
  measures "d43" distance of L16.start L16.end
  measures "d44" distance of L16.end L17.end
  measures "d45" distance of L0 L22
  measures "d46" distance of L1 L23
extrude "Extrude5" add sketch "Layout" along normal blind 1.9 contours L20 L21 L22 L23 | L24 L25 L26 L27 makes body 1 at (7.5333, 4.6, 0.6333) makes body 2 at (8.5667, -3.1, 0.6333)
extrude "Extrude1" add sketch "Layout" against normal blind 1.6 separate body contours L0 L1 L2 L3 L6 L7 L8 | L3 L6 L7 L8 L9 | L10 L11 L14 L15 | L12 L16 L17 L19 | L12 L17 L18 L19 | A0 | L20 L21 L22 L23 | L24 L25 L26 L27 makes body 3
hole "Hole1" at (-15.33, -7.73, 0) at (-12.79, -7.73, 0) at (-10.25, -7.73, 0) at (-7.71, -7.73, 0) at (-5.17, -7.73, 0) at (-2.63, -7.73, 0) at (-0.09, -7.73, 0) at (2.45, -7.73, 0) at (4.99, -7.73, 0) at (7.53, -7.73, 0) at (10.07, -7.73, 0) at (12.61, -7.73, 0) at (15.33, -6.35, 0) at (15.33, -3.81, 0) at (15.33, -1.27, 0) at (15.33, 1.27, 0) at (15.33, 3.81, 0) at (15.33, 6.35, 0) at (12.61, 7.73, 0) at (10.07, 7.73, 0) at (7.53, 7.73, 0) at (4.99, 7.73, 0) at (2.45, 7.73, 0) at (-0.09, 7.73, 0) at (-2.63, 7.73, 0) at (-5.17, 7.73, 0) at (-7.71, 7.73, 0) at (-10.25, 7.73, 0) at (-12.79, 7.73, 0) at (-15.33, 7.73, 0) direction (0, 0, -1) diameter 1 end up to surface (1.6 mm away) bodies 3
extrude "Extrude2" add sketch "Layout" along normal blind 2 separate body contours L10 L11 L14 L15 makes body 4
extrude "Extrude3" add sketch "Layout" along normal blind 1.5 separate body contours L3 L6 L7 L8 L9 | A0 makes body 5
extrude "Extrude4" add sketch "Layout" along normal blind 1 from surface at 1.5 separate body contours A0 makes body 6
fillet "Fillet1" radius 0.5 1 edges at (-15.3154, -0.452, 2.5) on bodies 6
fillet "Fillet2" radius 0.5 4 edges at (-5.3665, 2.3335, 2) (-0.6996, 2.3335, 2) (-5.3665, -2.3335, 2) (-0.6996, -2.3335, 2) on bodies 4 5
fillet "Fillet2" radius 0.5 12 edges at (1.6338, 0, 1) (-3.0331, -4.6669, 1) (-7.7, 0, 1) (-3.0331, 4.6669, 1) (-14.15, -2.45, 1.5) (-16.6, -2.45, 0.75) (-16.6, 2.45, 0.75) (-14.15, 2.45, 1.5) (-16.6, 0, 1.5) (-11.7, 0, 1.5) (-11.7, -2.45, 0.75) (-11.7, 2.45, 0.75) on bodies 4 5
extrude "Extrude6" add sketch "Layout" along normal blind 1.3 separate body contours L12 L16 L17 L19 | L12 L17 L18 L19 makes body 7
copy_body "Body->Comp1" bodies 1 removing the originals makes body 8 in component "Cap1"
copy_body "Body->Comp2" bodies 5 removing the originals makes body 9 in component "Reset Body"
copy_body "Body->Comp3" bodies 4 removing the originals makes body 10 in component "CPU"
copy_body "Body->Comp4" bodies 6 removing the originals makes body 11 in component "Reset Switch"
copy_body "Body->Comp5" bodies 7 removing the originals makes body 12 in component "Tx"
copy_body "Body->Comp6" bodies 2 removing the originals makes body 13 in component "Cap2"
copy_body "Body->Comp7" bodies 3 removing the originals makes body 14 in component "PCB"
component "Cap1" placed x (1, 0, 0) y (0, 1, 0) z (0, 0, 1) at (0, 0, 0)
component "Reset Body" placed x (1, 0, 0) y (0, 1, 0) z (0, 0, 1) at (0, 0, 0)
component "CPU" placed x (1, 0, 0) y (0, 1, 0) z (0, 0, 1) at (0, 0, 0)
component "Reset Switch" placed x (1, 0, 0) y (0, 1, 0) z (0, 0, 1) at (0, 0, 0)
component "Tx" placed x (1, 0, 0) y (0, 1, 0) z (0, 0, 1) at (0, 0, 0)
component "Cap2" placed x (1, 0, 0) y (0, 1, 0) z (0, 0, 1) at (0, 0, 0)
component "PCB" placed x (1, 0, 0) y (0, 1, 0) z (0, 0, 1) at (0, 0, 0)
named bodies: "PCB", "CPU", "Reset Body", "Reset Switch", "Cap1", "Cap2", "Tx"

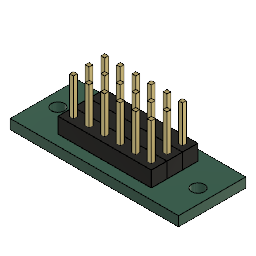
design "Servo Block"
Autodesk Fusion 360 part; units mm, degrees
sketch "PCB" plane through (0, 0, 0) normal (0, 0, 1) x (1, 0, 0)
  line L0 (-13.75, 5.5) -> (13.75, 5.5)
  line L1 (13.75, 5.5) -> (13.75, -5.5)
  line L2 (13.75, -5.5) -> (-13.75, -5.5)
  line L3 (-13.75, -5.5) -> (-13.75, 5.5)
  line L4 (-13.75, 5.5) -> (13.75, -5.5) construction
  line L5 (13.75, 5.5) -> (-13.75, -5.5) construction
  circle A0 centre (-11.43, 0) radius 1.05
  line L6 (0, 1.75) -> (0, 22.5)
  circle A1 centre (11.43, 0) radius 1.05
  line L7 (1.75, 0) -> (22.5, 0)
  point P0 (-6.35, -2.54)
  point P1 (-3.81, -2.54)
  point P2 (-1.27, -2.54)
  point P3 (-6.35, 0)
  point P4 (-3.81, 0)
  point P5 (-1.27, 0)
  point P6 (-6.35, 2.54)
  point P7 (-3.81, 2.54)
  point P8 (-1.27, 2.54)
  point P9 (1.27, -2.54)
  point P10 (1.27, 2.54)
  point P11 (3.81, -2.54)
  point P12 (6.35, -2.54)
  point P13 (6.35, 2.54)
  point P14 (1.27, 0)
  point P15 (3.81, 2.54)
  point P16 (6.35, 0)
  point P17 (3.81, 0)
  dimension "d5" = 2.1
  dimension "d9" = 2.54
  dimension "d10" = 2.54
  dimension "d11" = 2.54
  dimension "d12" = 27.5
  dimension "d18" = 5.08
  constraint horizontal L0
  constraint perpendicular L0 L1
  constraint parallel L0 L2
  constraint parallel L1 L3
  constraint coincident L4 origin
  constraint coincident L5 origin
  constraint symmetric A0 L6 A1
  constraint coincident L5 P0
  constraint coincident P3 L7
  constraint coincident A0.centre L7
  constraint symmetric L6 P0 P12
  constraint symmetric L6 P1 P11
  constraint symmetric L6 P2 P9
  constraint symmetric L6 P3 P16
  constraint symmetric L6 P4 P17
  constraint symmetric L6 P5 P14
  constraint symmetric L6 P6 P13
  constraint symmetric L6 P7 P15
  constraint symmetric L6 P8 P10
  measures "d5" diameter of A0
  measures "d11" distance of P2 P9
  measures "d12" distance of L0.start L0.end
  measures "d18" distance of A0.centre P3
extrude "Extrude1" add sketch "PCB" along normal blind 1.6 makes body 1
hole "Hole1" at (-6.35, 2.54, 0) at (-3.81, 2.54, 0) at (-1.27, 2.54, 0) at (1.27, 2.54, 0) at (3.81, 2.54, 0) at (6.35, 2.54, 0) at (6.35, 0, 0) at (3.81, 0, 0) at (1.27, 0, 0) at (1.27, -2.54, 0) at (-1.27, -2.54, 0) at (-6.35, -2.54, 0) at (-6.35, 0, 0) at (-3.81, -2.54, 0) at (3.81, -2.54, 0) at (-1.27, 0, 0) at (-3.81, 0, 0) at (6.35, -2.54, 0) direction (0, 0, 1) diameter 1 end up to surface (1.6 mm away) bodies 1
sketch "Header Pins" plane through (0, 0, 1.6) normal (0, 0, 1) x (-1, 0, 0)
  circle A0 centre (3.81, 0) radius 0.5
  circle A1 centre (-3.81, 2.54) radius 0.5
  circle A2 centre (6.35, 0) radius 0.5
  circle A3 centre (1.27, 2.54) radius 0.5
  circle A4 centre (-1.27, 0) radius 0.5
  circle A5 centre (-6.35, 0) radius 0.5
  circle A6 centre (-3.81, -2.54) radius 0.5 construction
  circle A7 centre (1.27, -2.54) radius 0.5 construction
  circle A8 centre (6.35, -2.54) radius 0.5 construction
  circle A9 centre (3.81, -2.54) radius 0.5 construction
  circle A10 centre (-1.27, -2.54) radius 0.5 construction
  circle A11 centre (-6.35, -2.54) radius 0.5 construction
  circle A12 centre (-3.81, 0) radius 0.5
  circle A13 centre (-1.27, 2.54) radius 0.5
  circle A14 centre (6.35, 2.54) radius 0.5
  circle A15 centre (3.81, 2.54) radius 0.5
  circle A16 centre (1.27, 0) radius 0.5
  circle A17 centre (-6.35, 2.54) radius 0.5
  circle A18 centre (-11.43, 0) radius 1.05
  circle A19 centre (11.43, 0) radius 1.05
  line L0 (13.75, 5.5) -> (-13.75, 5.5)
  line L1 (-13.75, 5.5) -> (-13.75, -5.5)
  line L2 (-13.75, -5.5) -> (13.75, -5.5)
  line L3 (13.75, -5.5) -> (13.75, 5.5)
  line L4 (7.62, -3.81) -> (-7.62, -3.81)
  line L5 (-7.62, -3.81) -> (-7.62, -1.27)
  line L6 (-7.62, -1.27) -> (7.62, -1.27)
  line L7 (7.62, -1.27) -> (7.62, -3.81)
  line L8 (6.675, -2.865) -> (6.025, -2.865)
  line L9 (6.025, -2.865) -> (6.025, -2.215)
  line L10 (6.025, -2.215) -> (6.675, -2.215)
  line L11 (6.675, -2.215) -> (6.675, -2.865)
  line L12 (6.675, -2.865) -> (6.025, -2.215) construction
  line L13 (6.025, -2.865) -> (6.675, -2.215) construction
  point P0 (6.35, -2.54)
  point P1 (-6.35, -2.54)
  point P2 (6.35, -2.54)
  dimension "d19" = 1.27
  dimension "d20" = 1.27
  dimension "d21" = 1.27
  dimension "d22" = 1.27
  dimension "d23" = 0.65
  dimension "d24" = 0.65
  constraint horizontal L4
  constraint vertical L5
  constraint horizontal L6
  constraint vertical L7
  constraint horizontal L8
  constraint perpendicular L8 L9
  constraint parallel L8 L10
  constraint parallel L9 L11
  constraint coincident L12 P2
  constraint coincident L13 P2
  constraint coincident P2 P0
  measures "d19" distance of L6 P2
  measures "d20" distance of L4 P2
  measures "d21" distance of L7 P2
  measures "d22" distance of L5 P1
  measures "d23" distance of L9.end L10.end
  measures "d24" distance of L8.end L9.end
extrude "Extrude2" add sketch "Header Pins" along normal blind 2.54 separate body contours L4 L5 L6 L7 | L8 L9 L10 L11 makes body 2
extrude "Extrude3" add sketch "Header Pins" along normal blind 8.54 and the other way blind 3 separate body contours L8 L9 L10 L11 makes body 3
copy_body "CutPasteBodies1" bodies 2 removing the originals makes body 4 in component "Header"
copy_body "CutPasteBodies2" bodies 3 removing the originals makes body 5 in component "Header"
pattern_linear "R-Pattern1" count 3 spacing 2.54 along (0, -1, 0) of bodies 4 makes body 6 at (-2.54, 1.27, 2.4467) makes body 7 at (2.54, -3.81, 2.4467) in component "Header"
pattern_linear "R-Pattern2" count 3 spacing 2.54 along (0, -1, 0) count 6 spacing 2.54 along (1, 0, 0) of bodies 5 makes body 8 at (-6.2417, 0.325, 6.2933) makes body 9 at (-6.2417, -2.215, 6.2933) makes body 10 at (-3.7017, 2.865, 6.2933) makes body 11 at (-3.7017, 0.325, 6.2933) makes body 12 at (-3.7017, -2.215, 6.2933) makes body 13 at (-1.1617, 2.865, 6.2933) makes body 14 at (-1.1617, 0.325, 6.2933) makes body 15 at (-1.1617, -2.215, 6.2933) makes body 16 at (1.3783, 2.865, 6.2933) makes body 17 at (1.3783, 0.325, 6.2933) makes body 18 at (1.3783, -2.215, 6.2933) makes body 19 at (3.9183, 2.865, 6.2933) makes body 20 at (3.9183, 0.325, 6.2933) makes body 21 at (3.9183, -2.215, 6.2933) makes body 22 at (6.4583, 2.865, 6.2933) makes body 23 at (6.4583, 0.325, 6.2933) makes body 24 at (6.4583, -2.215, 6.2933) in component "Header"
copy_body "Body->Comp1" bodies 1 removing the originals makes body 25 in component "PCB"
component "Header" placed x (1, 0, 0) y (0, 1, 0) z (0, 0, 1) at (0, 0, 0)
component "PCB" placed x (1, 0, 0) y (0, 1, 0) z (0, 0, 1) at (0, 0, 0)
equation "d20 = d19"
named bodies: "PCB", "Header Plastic", "Header Pin", "Header Plastic (1)", "Header Plastic (2)", "Header Pin (1)", "Header Pin (2)", "Header Pin (3)", "Header Pin (4)", "Header Pin (5)", "Header Pin (6)", "Header Pin (7)", "Header Pin (8)", "Header Pin (9)", "Header Pin (10)", "Header Pin (11)", "Header Pin (12)", "Header Pin (13)", "Header Pin (14)", "Header Pin (15)", "Header Pin (16)", "Header Pin (17)"
